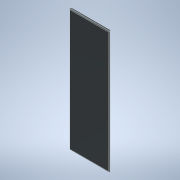
# Autodesk Inventor part: Base 2
Saved by Autodesk Inventor 2021 (Build 250183000, 183)
## iProperties
Created: 2021-06-29
Part Number: Base 2
Material: Iron, Gray
Document SubType Name: Modeling
Designer: Manojgouda K R
Density: 7.15 g/cm^3
Appearance: Iron Gray
Author: Manojgouda K R
Autodesk Inventor part; units mm, degrees
ref_plane "YZ Plane" through (0, 0, 0) normal (1, 0, 0) x (0, 1, 0)
ref_plane "XZ Plane" through (0, 0, 0) normal (0, 1, 0) x (-1, 0, 0)
ref_plane "XY Plane" through (0, 0, 0) normal (0, 0, 1) x (1, 0, 0)
sketch "Sketch1" plane through (0, 0, 0) normal (0, 0, 1) x (1, 0, 0)
  line L0 (0, 0) -> (10.42, 0)
  line L1 (10.42, 0) -> (10.42, -32)
  line L2 (10.42, -32) -> (0, -32)
  line L3 (0, -32) -> (0, 0)
  dimension "d0" = 10.42
  dimension "d1" = 32
  constraints: 8 end point, 2 parallel, 1 horizontal, 1 perpendicular
  measures "d0" distance of L1.end L2.end
  measures "d1" distance of L0.end L1.end
extrude "Extrusion1" add sketch "Sketch1" along normal blind 0.5
fillet "Fillet1" radius 0.2 6 edges at (5.21, 0, 0.5) (5.21, -32, 0.5) (10.42, -16, 0) (10.42, -16, 0.5) (0, -16, 0) (0, -16, 0.5)
body "Solid1"
